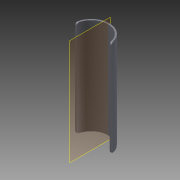
# Autodesk Inventor part: Soporte_Spool_001
Saved by Autodesk Inventor 2015 (Build 190159000, 159)
## iProperties
Created: 2013-09-02
Part Number: Soporte_Spool_001
Document SubType Name: Modeling
Designer: Estacion4
Density: 8.08 g/cm^3
Material: Stainless Steel
Mass: 61.4077 g
Surface Area: 105.782 cm^2
Volume: 7.59996 cm^3
Appearance: Steel
Author: Estacion4
Autodesk Inventor part; units mm, degrees
ref_plane "XZ Plane" through (0, 0, 0) normal (0, 1, 0) x (-1, 0, 0)
ref_plane "XY Plane" through (0, 0, 0) normal (0, 0, 1) x (1, 0, 0)
sketch "Boceto1" plane through (0, 0, 0) normal (0, 0, 1) x (1, 0, 0)
  circle A0 centre (0, 0) radius 18.5
  circle A1 centre (0, 0) radius 17
  line L0 (-18.3916, 2) -> (-16.8819, 2)
  line L1 (16.8819, 2) -> (18.3916, 2)
  dimension "d0" = 37
  dimension "d1" = 1.5
  dimension "d2" = 2
  constraints: 4 end point, 4 point on circle, 2 centre point, 2 coincident, 1 collinear, 1 horizontal, 1 horizontal alignment
  measures "d0" diameter of A0
  measures "d1" radial gap between concentric circles of A0 A1
  measures "d2" distance from line of L0 point (0, 0)
extrude "Extrusión1" add sketch "Boceto1" along normal blind 98 contours L1 A1 L0 A0 picked at (-2.8471, 17.6524)
fillet "Empalme1" radius 2.5 4 edges at (-17.6368, 2, 98) (17.6368, 2, 98) (-17.6368, 2, 0) (17.6368, 2, 0)
body "Solid1"
